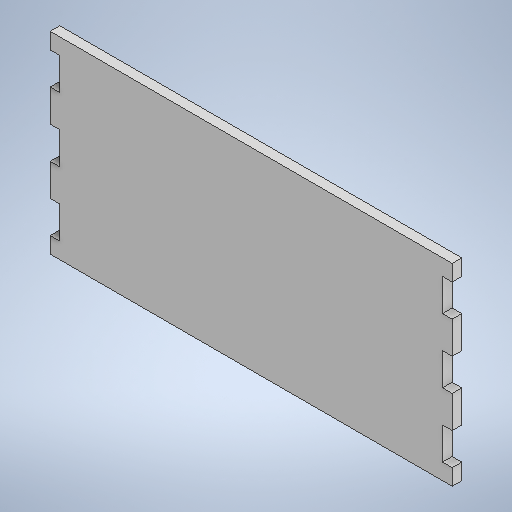
# Autodesk Inventor part: Archimedes Screw Border1
Saved by Autodesk Inventor 2025.3 (Build 293356000, 356)
## iProperties
Created: 2026-03-14
Part Number: Archimedes Screw Border1
Material: Generic
Document SubType Name: Modeling
Designer: ziada
Density: 1 g/cm^3
Appearance: Default
Author: ziada
Autodesk Inventor part; units mm, degrees
ref_plane "YZ Plane" through (0, 0, 0) normal (1, 0, 0) x (0, 1, 0)
ref_plane "XZ Plane" through (0, 0, 0) normal (0, 1, 0) x (-1, 0, 0)
ref_plane "XY Plane" through (0, 0, 0) normal (0, 0, 1) x (1, 0, 0)
sketch "Sketch1" plane through (0, 0, 0) normal (0, 0, 1) x (1, 0, 0)
  line L0 (0, 0) -> (0, 120)
  circle A0 centre (80, 60) radius 50
  line L1 (0, 0) -> (150, 0)
  line L2 (150, 120) -> (0, 120)
  line L3 (0, 120) -> (0, 110)
  line L4 (0, 110) -> (5, 110)
  line L5 (5, 110) -> (5, 90)
  line L6 (5, 90) -> (0, 90)
  line L7 (0, 90) -> (0, 70)
  line L8 (0, 70) -> (5, 70)
  line L9 (5, 70) -> (5, 50)
  line L10 (5, 50) -> (0, 50)
  line L11 (0, 50) -> (0, 30)
  line L12 (0, 30) -> (5, 30)
  line L13 (5, 30) -> (5, 10)
  line L14 (5, 10) -> (0, 10)
  line L15 (0, 120) -> (-50, 120)
  line L16 (-50, 120) -> (-50, 110)
  line L17 (-50, 110) -> (-44, 110)
  line L18 (-44, 110) -> (-44, 90)
  line L19 (-44, 90) -> (-50, 90)
  line L20 (-50, 90) -> (-50, 70)
  line L21 (-50, 70) -> (-44, 70)
  line L22 (-44, 70) -> (-44, 50)
  line L23 (-44, 50) -> (-50, 50)
  line L24 (-50, 50) -> (-50, 30)
  line L25 (-50, 30) -> (-44, 30)
  line L26 (-44, 30) -> (-44, 10)
  line L27 (-44, 10) -> (-50, 10)
  line L28 (-50, 10) -> (-50, 0)
  line L29 (-50, 0) -> (0, 0)
  line L30 (150, 115) -> (145, 115)
  line L31 (145, 115) -> (145, 95)
  line L32 (150, 120) -> (200, 120)
  line L33 (200, 120) -> (200, 110)
  line L34 (200, 110) -> (194, 110)
  line L35 (194, 110) -> (194, 90)
  line L36 (194, 90) -> (200, 90)
  line L37 (200, 90) -> (200, 70)
  line L38 (200, 70) -> (194, 70)
  line L39 (194, 70) -> (194, 50)
  line L40 (194, 50) -> (200, 50)
  line L41 (200, 50) -> (200, 30)
  line L42 (200, 30) -> (194, 30)
  line L43 (194, 30) -> (194, 10)
  line L44 (194, 10) -> (200, 10)
  line L45 (200, 10) -> (200, 0)
  line L46 (200, 0) -> (150, 0)
  line L47 (150, 120) -> (150, 0)
  line L48 (145, 95) -> (150, 95)
  line L49 (150, 95) -> (150, 90)
  line L50 (150, 90) -> (145, 90)
  line L51 (145, 90) -> (145, 70)
  line L52 (145, 70) -> (150, 70)
  line L53 (0, 120) -> (0, 125)
  line L54 (150, 125) -> (150, 120)
  line L55 (0, 125) -> (10, 125)
  line L56 (10, 125) -> (10, 120)
  line L57 (10, 120) -> (30, 120)
  line L58 (30, 120) -> (30, 125)
  line L59 (30, 125) -> (50, 125)
  line L60 (50, 125) -> (50, 120)
  line L61 (50, 120) -> (70, 120)
  line L62 (70, 120) -> (70, 125)
  line L63 (70, 125) -> (90, 125)
  line L64 (90, 125) -> (90, 120)
  line L65 (90, 120) -> (110, 120)
  line L66 (110, 120) -> (110, 125)
  line L67 (110, 125) -> (130, 125)
  line L68 (130, 125) -> (130, 120)
  line L69 (130, 120) -> (140, 120)
  line L70 (140, 120) -> (140, 125)
  line L71 (140, 125) -> (150, 125)
  dimension "d12" = 100
  dimension "d13" = 120
  dimension "d14" = 150
  dimension "d17" = 80
  dimension "d18" = 60
  dimension "d19" = 10
  dimension "d20" = 5
  dimension "d21" = 20
  dimension "d22" = 20
  dimension "d23" = 5
  dimension "d24" = 20
  dimension "d25" = 20
  dimension "d26" = 20
  dimension "d38" = 50
  dimension "d39" = 10
  dimension "d40" = 6
  dimension "d41" = 5
  dimension "d42" = 5
  dimension "d43" = 50
  dimension "d44" = 6
  dimension "d45" = 5
  dimension "d46" = 20
  dimension "d47" = 20
  dimension "d48" = 5
  dimension "d51" = 10
  dimension "d52" = 20
  dimension "d53" = 20
  dimension "d54" = 20
  dimension "d55" = 20
  dimension "d56" = 20
  dimension "d57" = 20
  dimension "d58" = 10
  constraints: 142 end point, 39 point on line, 31 perpendicular, 8 vertical, 6 horizontal, 1 centre point, 1 parallel, 11 other
  measures "d12" diameter of A0
  measures "d13" distance of L0.start L0.end
  measures "d14" distance of L32.start L0.end
  measures "d17" distance from line of L0 A0.centre
  measures "d19" distance of L0.end L3.end
  measures "d20" distance of L3.end L4.end
  measures "d21" distance of L4.end L5.end
  measures "d22" distance of L6.end L7.end
  measures "d23" distance of L7.end L8.end
  measures "d24" distance of L8.end L9.end
  measures "d25" distance of L10.end L11.end
  measures "d26" distance of L12.end L13.end
  measures "d38" distance of L0.end L15.end
  measures "d39" distance of L15.end L16.end
  measures "d40" distance of L16.end L17.end
  measures "d41" distance of L32.start L30.start
  measures "d42" distance of L30.start L30.end
  measures "d43" distance of L32.start L32.end
  measures "d44" distance of L33.end L34.end
  measures "d45" distance between parallel lines of L50 L48
  measures "d46" distance of L50.end L51.end
  measures "d47" distance of L30.end L31.end
  measures "d48" distance of L0.end L53.end
  measures "d51" distance of L53.end L55.end
  measures "d52" distance of L56.end L57.end
  measures "d53" distance of L58.end L59.end
  measures "d54" distance of L60.end L61.end
  measures "d55" distance of L62.end L63.end
  measures "d56" distance of L64.end L65.end
  measures "d57" distance of L66.end L67.end
  measures "d58" distance of L68.end L69.end
extrude "Extrusion1" add sketch "Sketch1" against normal blind 6 contours L29 L28 L27 L26 L25 L24 L23 L22 L21 L20 L19 L18 L17 L16 L15 L0 | L0 L14 L13 L12 L10 L9 L8 L6 L5 L4 L2 L47 L30 L31 L48 L50 L51 L52 L1 | L0 L12 L13 L14 | L47 L32 L33 L34 L35 L36 L37 L38 L39 L40 L41 L42 L43 L44 L45 L46 | L52 L51 L50 L47 | L0 L8 L9 L10 | L48 L31 L30 L47 | L0 L4 L5 L6 | A0
body "Solid1"
